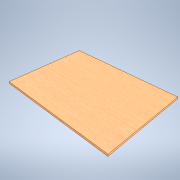
# Autodesk Inventor part: Base
Saved by Autodesk Inventor 2021.2 (Build 252289000, 289)
## iProperties
Created: 2021-03-19
Part Number: Base
Material: Wood (Cherry)
Document SubType Name: Modeling
Designer: 443201246
Density: 0.63 g/cm^3
Appearance: Cherry - Natural Low Gloss
Author: 443201246
Autodesk Inventor part; units mm, degrees
ref_plane "YZ Plane" through (0, 0, 0) normal (1, 0, 0) x (0, 1, 0)
ref_plane "XZ Plane" through (0, 0, 0) normal (0, 1, 0) x (-1, 0, 0)
ref_plane "XY Plane" through (0, 0, 0) normal (0, 0, 1) x (1, 0, 0)
sketch "Sketch1" plane through (0, 0, 0) normal (0, 1, 0) x (-1, 0, 0)
  line L0 (82, 59.5) -> (-82, 59.5)
  line L1 (-82, 59.5) -> (-82, -59.5)
  line L2 (-82, -59.5) -> (82, -59.5)
  line L3 (82, -59.5) -> (82, 59.5)
  line L4 (82, 59.5) -> (-82, -59.5) construction
  line L5 (-82, 59.5) -> (82, -59.5) construction
  point P0 (0, 0)
  dimension "d0" = 164
  dimension "d1" = 119
  constraints: 12 end point, 2 midpoint, 2 parallel, 1 horizontal, 1 perpendicular
  measures "d0" distance of L2.end L1.end
  measures "d1" distance of L1.end L0.end
extrude "Extrusion1" add sketch "Sketch1" against normal blind 3
body "Solid1"
